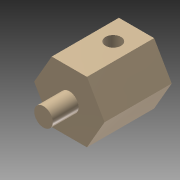
# Autodesk Inventor part: Hub_Hex_12mm
Saved by Autodesk Inventor 2014 SP1 (Build 180222100, 222)
## iProperties
Created: 2015-04-18
Part Number: Hub_Hex_12mm
Material: Polyethylene, Low Density
Document SubType Name: Modeling
Designer: david
Density: 0.894 g/cm^3
Appearance: Smooth - Off-White
Mass: 1.307 g
Surface Area: 10.015 cm^2
Volume: 1.46197 cm^3
Author: david
Autodesk Inventor part; units mm, degrees
ref_plane "YZ Plane" through (0, 0, 0) normal (1, 0, 0) x (0, 1, 0)
ref_plane "XZ Plane" through (0, 0, 0) normal (0, 1, 0) x (-1, 0, 0)
ref_plane "XY Plane" through (0, 0, 0) normal (0, 0, 1) x (1, 0, 0)
sketch "Sketch1" plane through (0, 0, 0) normal (0, 1, 0) x (-1, 0, 0)
  line L0 (6.8127, 0) -> (3.4064, -5.9)
  line L1 (3.4064, -5.9) -> (-3.4064, -5.9)
  line L2 (-3.4064, -5.9) -> (-6.8127, 0)
  line L3 (-6.8127, 0) -> (-3.4064, 5.9)
  line L4 (-3.4064, 5.9) -> (3.4064, 5.9)
  line L5 (3.4064, 5.9) -> (6.8127, 0)
  line L6 (0, 0) -> (25.8005, 0) construction
  dimension "d0" = 11.8
  constraints: 14 end point, 1 coincident, 1 horizontal, 1 point on line, 13 other
  measures "d0" distance between parallel lines of L1 L4
extrude "Extrusion1" add sketch "Sketch1" along normal blind 13
sketch "Sketch2" plane through (0, 13, 0) normal (0, 1, 0) x (1, 0, 0)
  line L0 (3.4064, 5.9) -> (-3.4064, 5.9) projected
  line L1 (-1.8439, 1.2) -> (1.8439, 1.2)
  line L2 (-1.8439, -1.2) -> (1.8439, -1.2)
  arc A0 (-1.8439, 1.2) -> (-1.8439, -1.2) centre (0, 0) ccw
  arc A1 (1.8439, -1.2) -> (1.8439, 1.2) centre (0, 0) ccw
  dimension "d4" = 2.4
  dimension "d5" = 2.2
  dimension "d6" = 2.2
  constraints: 4 end point, 4 point on circle, 3 parallel, 2 centre point, 1 coincident
  measures "d4" distance between parallel lines of L2 L1
  measures "d5" radius of A0
  measures "d6" radius of A1
extrude "Extrusion2" cut sketch "Sketch2" against normal blind 9
sketch "Sketch3" plane through (0, 0, 0) normal (0, -1, 0) x (1, 0, 0)
  circle A0 centre (0, 0) radius 1.8
  dimension "d9" = 3.6
  constraints: 1 centre point, 1 coincident
  measures "d9" diameter of A0
extrude "Extrusion3" add sketch "Sketch3" along normal blind 5
sketch "Sketch4" plane through (-3.4064, 0, 5.9) normal (0, 0, 1) x (1, 0, 0)
  line L0 (0, 13) -> (6.8127, 13) projected
  line L1 (0, 0) -> (0, 13) projected
  line L2 (3.4064, 0) -> (3.4064, 24.8022) construction
  circle A0 centre (3.4064, 8.5) radius 1.5
  dimension "d12" = 3
  dimension "d13" = 4.5
  constraints: 2 end point, 1 centre point, 1 parallel, 1 point on line
  measures "d12" diameter of A0
  measures "d13" distance from line of L0 A0.centre
extrude "Extrusion4" cut sketch "Sketch4" against normal through all
equation "\"Plastic_Reduction_Margin\" = 0.2"
body "Solid1"
